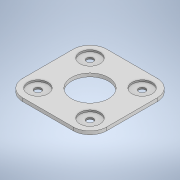
# Autodesk Inventor part: NEMA17_FacePlate
Saved by Autodesk Inventor 2021 (Build 250183000, 183)
## iProperties
Created: 2021-11-02
Part Number: NEMA17_FacePlate
Material: Generic
Document SubType Name: Modeling
Designer: Jorian Brusind
Density: 1 g/cm^3
Appearance: Default
Author: Jorian Brusind
Autodesk Inventor part; units mm, degrees
ref_plane "YZ Plane" through (0, 0, 0) normal (1, 0, 0) x (0, 1, 0)
ref_plane "XZ Plane" through (0, 0, 0) normal (0, 1, 0) x (-1, 0, 0)
ref_plane "XY Plane" through (0, 0, 0) normal (0, 0, 1) x (1, 0, 0)
sketch "Sketch1" plane through (0, 0, 0) normal (0, 1, 0) x (-1, 0, 0)
  line L0 (0, 0) -> (50, 0)
  line L1 (50, 0) -> (50, -50)
  line L2 (50, -50) -> (0, -50)
  line L3 (0, -50) -> (0, 0)
  circle A0 centre (40.5, -9.5) radius 2
  circle A1 centre (25, -25) radius 11
  circle A2 centre (40.5, -40.5) radius 2
  circle A3 centre (9.5, -9.5) radius 2
  circle A4 centre (9.5, -40.5) radius 2
  dimension "d0" = 50
  dimension "d1" = 50
  dimension "d2" = 4
  dimension "d3" = 9.5
  dimension "d4" = 9.5
  dimension "d5" = 22
  dimension "d6" = 25
  dimension "d7" = 25
  dimension "d10" = 31
  dimension "d13" = 31
  constraints: 8 end point, 5 centre point, 2 horizontal, 2 parallel, 1 perpendicular, 1 vertical, 6 other
  measures "d0" distance of L1.end L2.end
  measures "d1" distance of L0.end L1.end
  measures "d2" diameter of A0
  measures "d3" distance from line of L1 A0.centre
  measures "d4" distance from line of L0 A0.centre
  measures "d5" diameter of A1
  measures "d6" distance from line of L1 A1.centre
  measures "d7" distance from line of L2 A1.centre
  measures "d10" distance of A0.centre A2.centre
  measures "d13" distance of A0.centre A3.centre
extrude "Extrusion1" add sketch "Sketch1" along normal blind 2
fillet "Fillet1" radius 10 4 edges at (0, 1, -50) (0, 1, 0) (-50, 1, -50) (-50, 1, 0)
sketch "Sketch2" plane through (0, 2, 0) normal (0, 1, 0) x (1, 0, 0)
  circle A0 centre (-40.5, 9.5) radius 2 projected
  circle A1 centre (-40.5, 9.5) radius 6
  point P0 (0, 0)
  dimension "d19" = 12
  constraints: 1 centre point, 1 coincident
  measures "d19" diameter of A1
extrude "Extrusion2" cut sketch "Sketch2" against normal blind 1
pattern_linear "Rectangular Pattern1" count 2 spacing 31 along (1, 0, 0) count 2 spacing 31 along (0, 0, -1) of "Extrusion2"
body "Solid1"
